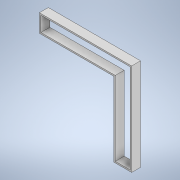
# Autodesk Inventor part: 축 케이스
Saved by Autodesk Inventor 2022 (Build 260153000, 153)
## iProperties
Created: 2022-10-28
Part Number: 축 케이스
Material: 일반
Document SubType Name: Modeling
Designer: whdls
Density: 1 g/cm^3
Appearance: 기본값
Author: whdls
Autodesk Inventor part; units mm, degrees
ref_plane "YZ Plane" through (0, 0, 0) normal (1, 0, 0) x (0, 1, 0)
ref_plane "XZ Plane" through (0, 0, 0) normal (0, 1, 0) x (-1, 0, 0)
ref_plane "XY Plane" through (0, 0, 0) normal (0, 0, 1) x (1, 0, 0)
sketch "스케치1" plane through (0, 0, 0) normal (0, 0, 1) x (1, 0, 0)
  line L0 (-25, 5) -> (5, 5)
  line L1 (0, 0) -> (-25, 0)
  line L2 (-25, 0) -> (-25, 5)
  line L3 (5, 5) -> (5, 5)
  line L4 (5, 5) -> (5, -25)
  line L5 (5, -25) -> (0, -25)
  line L6 (0, -25) -> (0, 0)
  line L7 (-25.5, 5.5) -> (0.0277, 5.5)
  line L8 (0, 0) -> (0, -0.5)
  line L9 (-0.5, -0.5) -> (-25.5, -0.5)
  line L10 (-25.5, -0.5) -> (-25.5, 5.5)
  line L11 (0.0277, 5.5) -> (5.5, 5.5)
  line L12 (5.5, 5.5) -> (5.5, -25.5)
  line L13 (5.5, -25.5) -> (-0.5, -25.5)
  line L14 (-0.5, -25.5) -> (-0.5, -0.5)
  point P0 (0, 0)
  dimension "d0" = 5
  dimension "d1" = 5
  dimension "d2" = 30
  dimension "d3" = 30
  dimension "d4" = 25
  dimension "d5" = 25
  dimension "d6" = 6
  dimension "d7" = 0.5
  dimension "d8" = 25.5
  dimension "d9" = 0.5
  dimension "d10" = 25.5
  dimension "d11" = 0.5
  constraints: 30 end point, 6 parallel, 4 horizontal, 4 perpendicular, 1 coincident, 1 point on line
  measures "d0" distance of L1.end L0.start
  measures "d1" distance of L4.end L5.end
  measures "d2" distance of L0.start L0.end
  measures "d3" distance of L3.end L4.end
  measures "d4" distance of L1.start L1.end
  measures "d5" distance of L1.start L5.end
  measures "d6" distance of L9.end L7.start
  measures "d7" distance between parallel lines of L1 L9
  measures "d8" distance between parallel lines of L6 L10
  measures "d9" distance between parallel lines of L12 L4
  measures "d10" distance between parallel lines of L1 L13
  measures "d11" distance between parallel lines of L6 L14
extrude "돌출1" add sketch "스케치1" along normal blind 3
